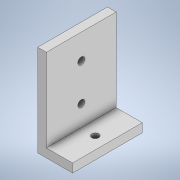
# Autodesk Inventor part: AutoCad Part3
Saved by Autodesk Inventor 2021 (Build 250183000, 183)
## iProperties
Created: 2024-01-19
Part Number: AutoCad Part3
Material: Generic
Document SubType Name: Modeling
Designer: Kumar Sanklap
Density: 1 g/cm^3
Appearance: Default
Author: Kumar Sanklap
Autodesk Inventor part; units mm, degrees
ref_plane "YZ Plane" through (0, 0, 0) normal (1, 0, 0) x (0, 1, 0)
ref_plane "XZ Plane" through (0, 0, 0) normal (0, 1, 0) x (-1, 0, 0)
ref_plane "XY Plane" through (0, 0, 0) normal (0, 0, 1) x (1, 0, 0)
sketch "Sketch1" plane through (0, 0, 0) normal (0, 0, 1) x (1, 0, 0)
  line L0 (0, 0) -> (0, 105)
  line L1 (0, 105) -> (10, 105)
  line L2 (10, 105) -> (10, 10)
  line L3 (10, 10) -> (40, 10)
  line L4 (40, 10) -> (40, 0)
  line L5 (40, 0) -> (0, 0)
  dimension "d0" = 105
  dimension "d1" = 10
  dimension "d2" = 95
  dimension "d3" = 30
  dimension "d4" = 10
  dimension "d5" = 40
  constraints: 12 end point, 2 horizontal, 2 perpendicular, 1 vertical
  measures "d0" distance of L0.start L0.end
  measures "d1" distance of L0.end L1.end
  measures "d2" distance of L1.end L2.end
  measures "d3" distance of L2.end L3.end
  measures "d4" distance of L3.end L4.end
  measures "d5" distance of L4.end L0.start
extrude "Extrusion1" add sketch "Sketch1" along normal blind 80
sketch "Sketch2" plane through (0, 0, 0) normal (-1, 0, 0) x (0, 0, 1)
  circle A0 centre (40, 34) radius 4
  point P0 (0, 0)
  dimension "d8" = 8
  constraints: 1 centre point
  measures "d8" diameter of A0
extrude "Extrusion2" cut sketch "Sketch2" against normal blind 10
pattern_linear "Rectangular Pattern1" count 2 spacing 42.5 along (0, 1, 0) of "Extrusion2"
sketch "Sketch3" plane through (0, 0, 0) normal (0, -1, 0) x (1, 0, 0)
  circle A0 centre (26, 40) radius 4
  point P0 (0, 0)
  dimension "d14" = 8
  constraints: 1 centre point
  measures "d14" diameter of A0
extrude "Extrusion3" cut sketch "Sketch3" against normal blind 10
body "Solid1"
